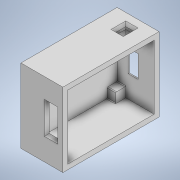
# Autodesk Inventor part: gehaeuse_wemos
Saved by Autodesk Inventor 2020 (Build 240168000, 168)
## iProperties
Created: 2020-05-23
Part Number: gehaeuse_wemos
Material: Generisch
Document SubType Name: Modeling
Designer: chris
Density: 1 g/cm^3
Appearance: Vorgabe
Author: chris
Autodesk Inventor part; units mm, degrees
ref_plane "YZ Plane" through (0, 0, 0) normal (1, 0, 0) x (0, 1, 0)
ref_plane "XZ Plane" through (0, 0, 0) normal (0, 1, 0) x (-1, 0, 0)
ref_plane "XY Plane" through (0, 0, 0) normal (0, 0, 1) x (1, 0, 0)
sketch "Skizze1" plane through (0, 0, 0) normal (1, 0, 0) x (0, 1, 0)
  line L0 (0, 0) -> (30, 0)
  line L1 (30, 0) -> (30, -39)
  line L2 (30, -39) -> (0, -39)
  line L3 (0, -39) -> (0, 0)
  dimension "d0" = 39
  dimension "d1" = 30
  constraints: 8 end point, 2 parallel, 1 horizontal, 1 perpendicular
  measures "d0" distance of L2.end L0.start
  measures "d1" distance of L0.start L0.end
extrude "Extrusion1" add sketch "Skizze1" along normal blind 17
shell "Wandung1" thickness 2 removed faces 1 at (17, 10, -13)
sketch "Skizze2" plane through (2, 2, -37) normal (1, 0, 0) x (0, 0, -1)
  line L0 (-35, 26) -> (-35, 0) projected
  line L1 (-35, 26) -> (-31, 26)
  line L2 (-31, 26) -> (-31, 22)
  line L3 (-31, 22) -> (-35, 22)
  line L4 (-35, 22) -> (-35, 26)
  line L5 (0, 26) -> (0, 0) projected
  line L6 (0, 26) -> (-4, 26)
  line L7 (-4, 26) -> (-4, 22)
  line L8 (-4, 22) -> (0, 22)
  line L9 (0, 22) -> (0, 26)
  line L10 (0, 0) -> (-4, 0)
  line L11 (-4, 0) -> (-4, 4)
  line L12 (-4, 4) -> (0, 4)
  line L13 (0, 4) -> (0, 0)
  line L14 (-35, 0) -> (0, 0) projected
  line L15 (-35, 0) -> (-31, 0)
  line L16 (-31, 0) -> (-31, 4)
  line L17 (-31, 4) -> (-35, 4)
  line L18 (-35, 4) -> (-35, 0)
  point P0 (-37, -2)
  point P1 (-35, 4)
  point P2 (-31, 0)
  point P3 (0, 4)
  point P4 (0, 22)
  dimension "d5" = 4
  dimension "d6" = 4
  dimension "d7" = 4
  dimension "d8" = 4
  constraints: 32 end point, 8 parallel, 4 horizontal, 4 perpendicular, 4 point on line
  measures "d5" distance of L2.end L3.end
  measures "d6" distance between parallel lines of L1 L3
  measures "d7" distance between parallel lines of L5 L7
  measures "d8" distance between parallel lines of L10 L12
extrude "Extrusion2" add sketch "Skizze2" along normal blind 3.5
fillet "Rundung1" radius 0.3 12 edges at (3.75, 24, -6) (3.75, 24, -2) (3.75, 28, -6) (3.75, 28, -33) (3.75, 24, -33) (3.75, 24, -37) (3.75, 6, -37) (3.75, 6, -33) (3.75, 2, -33) (3.75, 6, -2) (3.75, 6, -6) (3.75, 2, -6)
sketch "Skizze3" plane through (0, 0, -39) normal (0, 0, -1) x (-1, 0, 0)
  line L0 (-10.5, 20) -> (-6.5, 20)
  line L1 (-6.5, 20) -> (-6.5, 11)
  line L2 (-6.5, 11) -> (-10.5, 11)
  line L3 (-10.5, 11) -> (-10.5, 20)
  line L4 (0, 30) -> (-17, 30) projected
  line L5 (0, 0) -> (-17, 0) projected
  line L6 (0, 0) -> (0, 30) projected
  dimension "d12" = 9
  dimension "d13" = 4
  dimension "d15" = 11
  dimension "d16" = 6.5
  constraints: 8 end point, 2 parallel, 1 horizontal, 1 perpendicular
  measures "d12" distance between parallel lines of L2 L0
  measures "d13" distance between parallel lines of L1 L3
  measures "d15" distance between parallel lines of L5 L2
  measures "d16" distance between parallel lines of L6 L1
extrude "Extrusion3" cut sketch "Skizze3" against normal blind 3.5
sketch "Skizze4" plane through (0, 0, -39) normal (0, 0, -1) x (-1, 0, 0)
  line L0 (-13.5, 9) -> (-3.5, 9)
  line L1 (-3.5, 9) -> (-3.5, 22)
  line L2 (-3.5, 22) -> (-13.5, 22)
  line L3 (-13.5, 22) -> (-13.5, 9)
  line L4 (-10.5, 11) -> (-10.5, 20) projected
  line L5 (-6.5, 11) -> (-10.5, 11) projected
  point P0 (0, 0)
  dimension "d19" = 3
  dimension "d20" = 10
  dimension "d21" = 13
  dimension "d22" = 2
  constraints: 8 end point, 2 parallel, 1 horizontal, 1 perpendicular
  measures "d19" distance between parallel lines of L3 L4
  measures "d20" distance between parallel lines of L1 L3
  measures "d21" distance between parallel lines of L2 L0
  measures "d22" distance between parallel lines of L0 L5
extrude "Extrusion4" cut sketch "Skizze4" against normal blind 1.5
sketch "Skizze5" plane through (0, 0, 0) normal (0, 0, 1) x (1, 0, 0)
  line L0 (15, 22) -> (9.5, 22)
  line L1 (9.5, 22) -> (9.5, 9)
  line L2 (9.5, 9) -> (15, 9)
  line L3 (15, 9) -> (15, 22)
  line L4 (17, 30) -> (17, 0) projected
  line L5 (0, 30) -> (17, 30) projected
  point P0 (0, 0)
  dimension "d25" = 13
  dimension "d26" = 5.5
  dimension "d27" = 2
  dimension "d28" = 8
  constraints: 8 end point, 2 parallel, 1 horizontal, 1 perpendicular
  measures "d25" distance between parallel lines of L0 L2
  measures "d26" distance between parallel lines of L1 L3
  measures "d27" distance between parallel lines of L4 L3
  measures "d28" distance between parallel lines of L5 L0
extrude "Extrusion5" cut sketch "Skizze5" against normal blind 2
sketch "Skizze6" plane through (0, 30, 0) normal (0, 1, 0) x (1, 0, 0)
  line L0 (10.5, 31) -> (7.5, 31)
  line L1 (7.5, 31) -> (7.5, 35)
  line L2 (7.5, 35) -> (10.5, 35)
  line L3 (10.5, 35) -> (10.5, 31)
  line L4 (0, 39) -> (17, 39) projected
  line L5 (0, 39) -> (0, 0) projected
  dimension "d31" = 3
  dimension "d32" = 4
  dimension "d33" = 4
  dimension "d34" = 7.5
  constraints: 8 end point, 2 parallel, 1 horizontal, 1 perpendicular
  measures "d31" distance between parallel lines of L1 L3
  measures "d32" distance between parallel lines of L0 L2
  measures "d33" distance between parallel lines of L4 L2
  measures "d34" distance between parallel lines of L5 L1
extrude "Extrusion6" cut sketch "Skizze6" against normal blind 2
chamfer "Fase1" distance 1 angle 45 4 edges at (7.5, 30, -33) (9, 30, -31) (9, 30, -35) (10.5, 30, -33)
chamfer "Fase2" distance 1 angle 45 4 edges at (3.5, 15.5, -39) (8.5, 9, -39) (13.5, 15.5, -39) (8.5, 22, -39)
